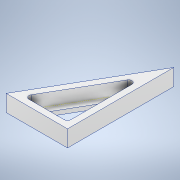
# Autodesk Inventor part: StaninaOpora.iam
Saved by Autodesk Inventor 2022 (Build 260153000, 153)
## iProperties
Created: 2023-08-15
Part Number: StaninaOpora.iam
Material: Aluminum 6061
Document SubType Name: Modeling
Designer: Kippi
Mass: 1259.99 g
Surface Area: 793.824 cm^2
Volume: 466.662 cm^3
Density: 2.7 g/cm^3
Appearance: Aluminum - Flat
Author: Kippi
Autodesk Inventor part; units mm, degrees
ref_plane "YZ Plane" through (0, 0, 0) normal (1, 0, 0) x (0, 1, 0)
ref_plane "XZ Plane" through (0, 0, 0) normal (0, 1, 0) x (-1, 0, 0)
ref_plane "XY Plane" through (0, 0, 0) normal (0, 0, 1) x (1, 0, 0)
sketch "Sketch1" plane through (0, 0, 0) normal (0, 1, 0) x (-1, 0, 0)
  line L0 (137.5, 125) -> (-10.3, 125)
  line L1 (-10.3, 125) -> (-10.3, -131)
  line L2 (-10.3, -131) -> (137.5, -131)
  line L3 (137.5, -131) -> (137.5, 125)
  line L4 (137.5, 125) -> (-10.3, -131)
  point P0 (0, 0)
  dimension "d0" = 256
  dimension "d1" = 147.8
  dimension "d7" = 30
  constraints: 10 end point, 2 parallel, 1 horizontal, 1 perpendicular
  measures "d0" distance of L0.end L1.end
  measures "d1" distance of L0.start L0.end
extrude "Extrusion1" add sketch "Sketch1" along normal blind 40 contours L4 L1 L0
sketch "Sketch2" plane through (0, 40, 0) normal (0, 1, 0) x (1, 0, 0)
  line L0 (-137.5, -125) -> (10.3, -125) construction
  line L1 (10.3, -125) -> (10.3, 131) construction
  line L2 (10.3, 131) -> (-137.5, -125) construction
  line L3 (-137.5, -125) -> (10.3, -125) construction
  line L4 (10.3, -125) -> (10.3, 131) construction
  line L5 (10.3, 131) -> (-137.5, -125) construction
  line L6 (-111.5194, -110) -> (-4.7, -110)
  line L7 (-4.7, -110) -> (-4.7, 75.0187)
  line L8 (-4.7, 75.0187) -> (-111.5194, -110)
  point P0 (0, 0)
  dimension "d4" = 15
  constraints: 6 end point, 2 other
  measures "d4" distance between parallel lines of L2 L8
extrude "Extrusion2" cut sketch "Sketch2" against normal blind 30
sketch "Sketch3" plane through (0, 10, 0) normal (0, 1, 0) x (1, 0, 0)
  line L0 (-4.7, 75.0187) -> (-4.7, -110) construction
  line L1 (-111.5194, -110) -> (-4.7, 75.0187) construction
  line L2 (-4.7, -110) -> (-111.5194, -110) construction
  point P0 (0, 0)
sketch "Sketch4" plane through (0, 10, 0) normal (0, 1, 0) x (1, 0, 0)
  line L0 (-4.7, 75.0187) -> (-4.7, -110) construction
  line L1 (-111.5194, -110) -> (-4.7, 75.0187) construction
  line L2 (-4.7, -110) -> (-111.5194, -110) construction
  line L3 (-4.7, 75.0187) -> (-4.7, -110) construction
  line L4 (-111.5194, -110) -> (-4.7, 75.0187) construction
  line L5 (-4.7, -110) -> (-111.5194, -110) construction
  line L6 (-19.7, 19.0374) -> (-19.7, -95)
  line L7 (-19.7, -95) -> (-85.5388, -95)
  line L8 (-85.5388, -95) -> (-19.7, 19.0374)
  point P0 (0, 0)
  dimension "d9" = 15
  constraints: 6 end point, 2 other
  measures "d9" distance between parallel lines of L6 L0
extrude "Extrusion3" cut sketch "Sketch4" against normal blind 30
fillet "Fillet2" radius 8 6 edges at (-4.7, 25, -75.0187) (-111.5194, 25, 110) (-4.7, 25, 110) (-19.7, 5, 95) (-85.5388, 5, 95) (-19.7, 5, -19.0374)
body "Solid1"
